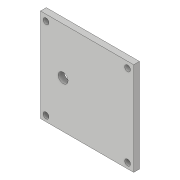
# Autodesk Inventor part: 2 nd part of capping syStem
Saved by Autodesk Inventor 2019 (Build 230136000, 136)
## iProperties
Created: 2019-10-13
Part Number: 2 nd part of capping syStem
Material: Generic
Document SubType Name: Modeling
Designer: Admin
Density: 1 g/cm^3
Appearance: Default
Author: Admin
Autodesk Inventor part; units mm, degrees
ref_plane "YZ Plane" through (0, 0, 0) normal (1, 0, 0) x (0, 1, 0)
ref_plane "XZ Plane" through (0, 0, 0) normal (0, 1, 0) x (-1, 0, 0)
ref_plane "XY Plane" through (0, 0, 0) normal (0, 0, 1) x (1, 0, 0)
sketch "Sketch1" plane through (0, 0, 0) normal (0, 0, 1) x (1, 0, 0)
  line L0 (0, 0) -> (160, 0)
  line L1 (160, 0) -> (160, 160)
  line L2 (160, 160) -> (0, 160)
  line L3 (0, 160) -> (0, 0)
  dimension "d0" = 160
  dimension "d1" = 160
  constraints: 8 end point, 2 parallel, 1 horizontal, 1 perpendicular
  measures "d0" distance of L2.end L1.end
  measures "d1" distance of L1.end L0.end
extrude "Extrusion1" add sketch "Sketch1" along normal blind 10
sketch "Sketch2" plane through (0, 0, 10) normal (0, 0, 1) x (1, 0, 0)
  line L0 (0, 0) -> (160, 0) projected
  line L1 (0, 0) -> (10, 0)
  line L2 (10, 0) -> (10, 150)
  line L3 (10, 150) -> (150, 150)
  dimension "d4" = 10
  dimension "d5" = 150
  dimension "d6" = 140
  constraints: 6 end point, 2 perpendicular, 1 point on line
  measures "d4" distance of L0.start L1.end
  measures "d5" distance of L1.end L2.end
  measures "d6" distance of L2.end L3.end
sketch "Sketch3" plane through (0, 0, 10) normal (0, 0, 1) x (1, 0, 0)
  line L0 (150.8125, 150.8125) -> (150.8125, 10.8125)
  line L1 (150.8125, 10.8125) -> (10.8125, 10.8125)
  line L2 (10.8125, 10.8125) -> (10.8125, 80.8125)
  line L3 (10.8125, 80.8125) -> (150.8125, 80.8125)
  circle A0 centre (10.8125, 150.8125) radius 5
  circle A1 centre (150.8125, 150.8125) radius 5
  circle A2 centre (150.8125, 10.8125) radius 5
  circle A3 centre (10.8125, 10.8125) radius 5
  point P0 (0, 0)
  dimension "d7" = 140
  dimension "d8" = 140
  dimension "d9" = 70
  dimension "d10" = 140
  dimension "d11" = 10
  dimension "d12" = 10
  dimension "d14" = 10
  dimension "d15" = 10
  constraints: 8 end point, 4 centre point, 3 coincident, 2 perpendicular, 1 midpoint, 1 vertical
  measures "d7" distance of L0.start L0.end
  measures "d8" distance of L0.end L1.end
  measures "d9" distance of L1.end L2.end
  measures "d10" distance of L2.end L3.end
  measures "d11" diameter of A0
  measures "d12" diameter of A1
  measures "d14" diameter of A2
  measures "d15" diameter of A3
extrude "Extrusion2" [suppressed]
sketch "Sketch4" plane through (0, 0, 10) normal (0, 0, 1) x (1, 0, 0)
  line L0 (0, 160) -> (0, 0) projected
  line L1 (0, 80) -> (30, 80)
  line L2 (30, 80) -> (33, 80)
  line L3 (33, 80) -> (36.5125, 80)
  line L4 (36.5125, 80) -> (41.275, 80)
  circle A0 centre (38.8938, 80) radius 8.5
  dimension "d19" = 30
  dimension "d36" = 3
  dimension "d40" = 17
  constraints: 8 end point, 3 horizontal, 2 midpoint, 1 centre point
  measures "d19" distance of L1.start L1.end
  measures "d36" distance of L1.end L2.end
  measures "d40" diameter of A0
extrude "Extrusion3" cut sketch "Sketch4" against normal through all
sketch "Sketch5" plane through (0, 0, 10) normal (0, 0, 1) x (1, 0, 0)
  line L0 (0, 160.3375) -> (9.9943, 160)
  line L1 (160, 160) -> (0, 160) projected
  line L2 (9.9943, 160) -> (159.9943, 160)
  line L3 (159.9943, 160) -> (159.9943, 0)
  line L4 (159.9943, 0) -> (147.6375, 0)
  point P0 (0, 0)
  dimension "d23" = 10
  dimension "d24" = 150
  constraints: 8 end point, 2 point on line, 1 perpendicular
  measures "d23" distance of L0.start L0.end
  measures "d24" distance of L0.end L2.end
sketch "Sketch6" plane through (0, 0, 10) normal (0, 0, 1) x (1, 0, 0)
  line L0 (160, 160) -> (0, 160) projected
  line L1 (160, 160) -> (160, 150)
  line L2 (160, 0) -> (160, 160) projected
  line L3 (160, 150) -> (10, 150)
  line L4 (10, 150) -> (10, 10)
  line L5 (0, 0) -> (160, 0) projected
  dimension "d25" = 10
  dimension "d26" = 150
  dimension "d27" = 140
  constraints: 6 end point, 2 perpendicular, 1 point on line
  measures "d25" distance of L0.start L1.end
  measures "d26" distance of L1.end L3.end
  measures "d27" distance of L3.end L4.end
sketch "Sketch7" plane through (0, 0, 10) normal (0, 0, 1) x (1, 0, 0)
  line L0 (9.525, 9.525) -> (149.525, 9.525)
  line L1 (149.525, 9.525) -> (149.525, 149.525)
  circle A0 centre (9.525, 9.525) radius 5
  circle A1 centre (9.525, 149.525) radius 5
  circle A2 centre (149.525, 149.525) radius 5
  circle A3 centre (149.525, 9.525) radius 5
  point P0 (0, 0)
  dimension "d28" = 140
  dimension "d29" = 140
  dimension "d30" = 10
  dimension "d31" = 10
  dimension "d32" = 10
  dimension "d33" = 10
  constraints: 4 centre point, 4 end point, 3 coincident, 1 horizontal, 1 perpendicular
  measures "d28" distance of L0.start L0.end
  measures "d29" distance of L0.end L1.end
  measures "d30" diameter of A0
  measures "d31" diameter of A1
  measures "d32" diameter of A2
  measures "d33" diameter of A3
extrude "Extrusion4" cut sketch "Sketch7" against normal through all
body "Solid1"
